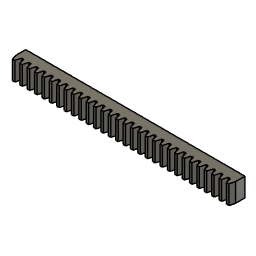
_Test Thread.e67c5d5b-8ed2-4406-8ac4-c447bfbe1a1b (Autodesk Fusion 360 design; units mm, degrees)
Autodesk Fusion 360 part; units mm, degrees
sketch "Sketch1" plane through (0, 0, 0) normal (0, 0, 1) x (1, 0, 0) in component "Component"
  line L0 (0, 0) -> (0.5819, 2.25)
  line L1 (1.6355, 2.25) -> (2.2173, 0)
  line L2 (0.5819, 2.25) -> (1.6355, 2.25)
  line L3 (0, 0) -> (0, -4)
  line L4 (0, -4) -> (2.2173, -4)
  line L5 (2.2173, -4) -> (2.2173, 0)
  line L6 (1.2753, 0) -> (100, 0)
  line L7 (0, 0, 0) -> (0, 0, 8)
sketch "Sketch2" plane through (0, 0, 0) normal (0, 0, 1) x (1, 0, 0) in component "Component"
  line L0 (0, 0) -> (93.3235, 0)
  line L1 (0, 0) -> (0, -4)
  line L2 (0, -4) -> (93.3235, -4)
  line L3 (93.3235, -4) -> (93.3235, 0)
sweep "Sweep1" add profiles "Sketch1" path "Sketch1" along L7 section 1 makes body 1 in component "Component"
pattern_path "PathPattern1" count 30 spacing 3.1416 from (1.2753, 0, 0) path "Sketch1" along L6 of "Sweep1" makes body 2 makes body 3 makes body 4 makes body 5 makes body 6 makes body 7 makes body 8 makes body 9 makes body 10 makes body 11 makes body 12 makes body 13 makes body 14 makes body 15 makes body 16 makes body 17 makes body 18 makes body 19 makes body 20 makes body 21 makes body 22 makes body 23 makes body 24 makes body 25 makes body 26 makes body 27 makes body 28 makes body 29 makes body 30 in component "Component"
extrude "Extrude1" add sketch "Sketch2" along normal blind 8 bodies 1 2 3 4 5 6 7 8 9 10 11 12 13 14 15 16 17 18 19 20 21 22 23 24 25 26 27 28 29 30 in component "Component"
move_body "Move1" bodies 1 to x (1, 0, 0) y (0, 0, 1) z (0, -1, 0) at (0, -4, 4) in component "Component"
sketch "Sketch3" plane through (0, 0, 0) normal (0, 0, 1) x (1, 0, 0) in component "Component"
  line L0 (0, 0) -> (50.8022, 0) construction
  line L1 (50.8022, 0) -> (50.8022, 3) construction
  line L2 (50.8022, 3) -> (0, 3) construction
  line L3 (0, 3) -> (0, 0) construction
  constraint perpendicular L0 L1
  constraint parallel L0 L2
  constraint parallel L1 L3
component "Component" placed x (1, 0, 0) y (0, 1, 0) z (0, 0, 1) at (0, 0, 0)
